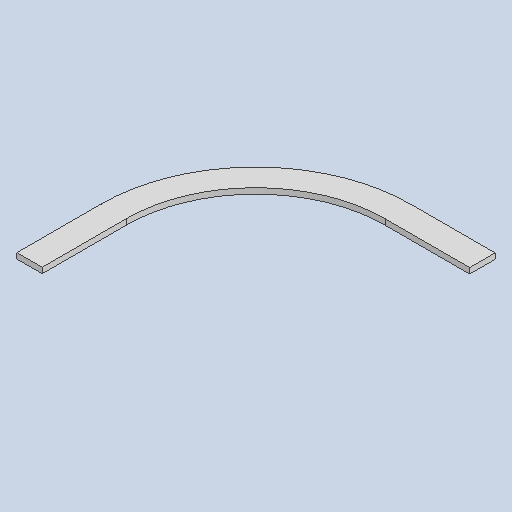
# Autodesk Inventor part: test1
Saved by Autodesk Inventor 2025 (Build 290162000, 162)
## iProperties
Created: 2025-04-20
Part Number: test1
Material: Generic
Document SubType Name: Sheet Metal
Designer: Pravoslav
Density: 1 g/cm^3
Sheet Metal Rule: Default_mm
Appearance: Default
Author: Pravoslav
Autodesk Inventor part; units mm, degrees
ref_plane "YZ Plane" through (0, 0, 0) normal (1, 0, 0) x (0, 1, 0)
ref_plane "XZ Plane" through (0, 0, 0) normal (0, 1, 0) x (-1, 0, 0)
ref_plane "XY Plane" through (0, 0, 0) normal (0, 0, 1) x (1, 0, 0)
sketch "Sketch1" plane through (0, 0, 0) normal (0, 1, 0) x (-1, 0, 0)
  circle A0 centre (0, 0) radius 55
  circle A1 centre (0, 0) radius 46
  line L0 (46, 0) -> (55.0071, 0)
  line L1 (55.0071, 0) -> (55.0071, 30)
  line L2 (55.0071, 30) -> (46, 30)
  line L3 (46, 30) -> (46, 0)
  line L4 (-0.2088, -45.9995) -> (-30.2088, -45.9995)
  line L5 (-30.2088, -45.9995) -> (-30.2088, -55.0484)
  line L6 (-30.2088, -55.0484) -> (-0.2088, -55.0484)
  line L7 (-0.2088, -55.0484) -> (-0.2088, -45.9995)
  point P0 (-22.8069, -50.0484)
  point P1 (50.0071, 22.8974)
  point P2 (-30.1503, -45.9995)
  point P3 (41, 28.6182)
  point P4 (55, 0)
  point P5 (-0.2088, -54.9996)
  dimension "d0" = 110
  dimension "d1" = 92
  dimension "d2" = 30
  dimension "d3" = 30
  constraints: 16 end point, 4 parallel, 2 centre point, 2 coincident, 2 horizontal, 2 perpendicular, 2 point on circle
  measures "d0" diameter of A0
  measures "d1" diameter of A1
  measures "d2" distance of L1.end L0.end
  measures "d3" distance of L6.end L5.end
extrude "Extrusion1" add sketch "Sketch1" along normal blind 2 contours L0 L3 L2 A0 | A0 L7 A1 L0 | A0 L2 L1 L0 | L7 L6 L5 L4 A0 | A0 L4 L7
equation "\"BendRadius\" = Thickness"
equation "\"BendReliefWidth\" = Thickness"
equation "\"BendReliefDepth\" = 0.5 * Thickness"
equation "\"CornerReliefSize\" = 4 * Thickness"
equation "\"MinimumRemnant\" = 2 * Thickness"
equation "\"TransitionRadius\" = BendRadius"
equation "\"JacobiRadiusSize\" = BendRadius"
equation "\"GapSize\" = Thickness"
equation "\"Thickness\" = 0.5"
body "Solid1"
